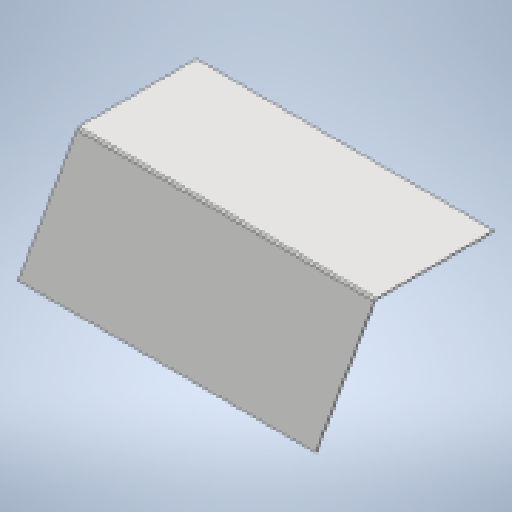
# Autodesk Inventor part: TRM 017 sheet in
Saved by Autodesk Inventor 2025 (Build 290162010, 162A)
## iProperties
Created: 2024-08-07
Part Number: TRM 017 sheet in
Material: AISI 304
Document SubType Name: Sheet Metal
Designer: pokla
Density: 8.02768 g/cm^3
Flat Pattern Width: 50 cm
Flat Pattern Length: 77.1162 cm
Flat Pattern Area: 3855.81 cm^2
Sheet Metal Rule: AISI304 2mm Die16
Sheet Metal Width: 500,000 mm
Sheet Metal Length: 771,162 mm
Sheet Metal Area: 385580,927 mm^2
Appearance: Default
Author: pokla
Autodesk Inventor part; units mm, degrees
ref_plane "YZ Plane" through (0, 0, 0) normal (1, 0, 0) x (0, 1, 0)
ref_plane "XZ Plane" through (0, 0, 0) normal (0, 1, 0) x (-1, 0, 0)
ref_plane "XY Plane" through (0, 0, 0) normal (0, 0, 1) x (1, 0, 0)
sketch "Sketch1" plane through (0, 0, 0) normal (0, 0, 1) x (1, 0, 0)
  line L0 (-250, -25) -> (250, -25)
  line L1 (250, -25) -> (250, 25)
  line L2 (250, 25) -> (-250, 25)
  line L3 (-250, 25) -> (-250, -25)
  line L4 (-250, -25) -> (250, 25) construction
  line L5 (250, -25) -> (-250, 25) construction
  point P0 (0, 0)
  dimension "d0" = 500
  dimension "d1" = 50
  measures "d0" distance of L2.end L1.end
  measures "d1" distance of L1.end L0.end
extrude "Plate1" add sketch "Sketch1" along normal blind 2
sketch "Sketch2" plane through (0, 0, 0) normal (0, 0, -1) x (-1, 0, 0)
  line L0 (-230, 5) -> (-30, 5) construction
  line L1 (-30, 5) -> (-30, -15) construction
  line L2 (-30, -15) -> (-230, -15) construction
  line L3 (-230, -15) -> (-230, 5) construction
  line L4 (-250, 25) -> (250, 25) projected
  line L5 (-250, -25) -> (-250, 25) projected
  point P0 (0, 0)
  point P1 (-48, 100)
  point P2 (250, 25)
  point P3 (-50, 98)
  dimension "d6" = 200
  dimension "d9" = 20
  dimension "d10" = 20
  dimension "d11" = 20
  constraints: 4 other
  measures "d6" distance of L0.start L0.end
  measures "d9" distance of L0.end L1.end
  measures "d11" length of L3
mark "Mark1"
sketch "Sketch3" plane through (-250, -23.1206, 1.316) normal (0, -0.9396926, 0.3420201) x (1, 0, 0)
  line L0 (500, 0) -> (0, 0)
  line L1 (0, 0) -> (0, -400)
  line L2 (0, -400) -> (500, -400)
  line L3 (500, -400) -> (500, 0)
  constraints: 6 end point, 1 horizontal, 1 perpendicular, 1 vertical
edge flange "Flange1" height 400 angle 70 thickness 2 bend radius 2.75 thickness toward (0, -0.9396926, 0.3420201) relief round relief width 2 relief depth 1 edges at (0, -25, 0) wall of the first edge with corners at (250, -23.1206, 1.316) (-250, -23.1206, 1.316) (-250, -159.9287, -374.5611) (250, -159.9287, -374.5611)
bend "Bend1"
corner "Corner1"
sketch "Sketch4" plane through (250, -159.9287, -372.5611) normal (0, 0, -1) x (-1, 0, 0)
  line L0 (500, 0) -> (0, 0)
  line L1 (0, 0) -> (0, -180)
  line L2 (0, -180) -> (500, -180)
  line L3 (500, -180) -> (500, 0)
  constraints: 6 end point, 1 horizontal, 1 perpendicular, 1 vertical
edge flange "Flange2" height 180 angle 70 thickness 2 bend radius 2.75 thickness toward (0, 0, -1) relief round relief width 2 relief depth 1 edges at (0, -161.8081, -373.877) wall of the first edge with corners at (-250, -159.9287, -372.5611) (250, -159.9287, -372.5611) (250, -339.9287, -372.5611) (-250, -339.9287, -372.5611)
bend "Bend2"
corner "Corner2"
sketch "Sketch5" plane through (250, -338.5145, -373.1469) normal (0, -0.7071068, -0.7071068) x (1, 0, 0)
  line L0 (-500, 0) -> (0, 0)
  line L1 (0, 0) -> (0, 100)
  line L2 (0, 100) -> (-500, 100)
  line L3 (-500, 100) -> (-500, 0)
  constraints: 6 end point, 1 horizontal, 1 perpendicular, 1 vertical
edge flange "Flange3" height 100 angle 45 thickness 2 bend radius 2.75 thickness toward (0, -0.7071068, -0.7071068) relief round relief width 2 relief depth 1 edges at (0, -339.9287, -372.5611) wall of the first edge with corners at (-250, -338.5145, -373.1469) (250, -338.5145, -373.1469) (250, -409.2251, -302.4362) (-250, -409.2251, -302.4362)
bend "Bend3"
corner "Corner3"
sketch "Sketch6" plane through (-250, -407.9396, -303.9683) normal (0, -0.6427876, 0.7660444) x (1, 0, 0)
  line L0 (500, 0) -> (0, 0)
  line L1 (0, 0) -> (0, -50)
  line L2 (0, -50) -> (500, -50)
  line L3 (500, -50) -> (500, 0)
  constraints: 6 end point, 1 horizontal, 1 perpendicular, 1 vertical
edge flange "Flange4" height 50 angle 85 thickness 2 bend radius 2.75 thickness toward (0, -0.6427876, 0.7660444) relief round relief width 2 relief depth 1 edges at (0, -410.6394, -303.8504) wall of the first edge with corners at (250, -407.9396, -303.9683) (-250, -407.9396, -303.9683) (-250, -446.2418, -336.1077) (250, -446.2418, -336.1077)
bend "Bend4"
corner "Corner4"
equation "\"d2\" = Thickness"
equation "\"d12\" = BendReliefWidth"
equation "\"d13\" = BendReliefDepth"
equation "\"d14\" = MinimumRemnant"
equation "\"d15\" = TransitionRadius"
equation "\"d18\" = BendRadius"
equation "\"d19\" = CornerReliefSize"
equation "\"d20\" = GapSize"
equation "\"d21\" = JacobiRadiusSize"
equation "\"d22\" = BendReliefWidth"
equation "\"d23\" = BendReliefDepth"
equation "\"d24\" = MinimumRemnant"
equation "\"d25\" = TransitionRadius"
equation "\"d28\" = BendRadius"
equation "\"d29\" = CornerReliefSize"
equation "\"d30\" = GapSize"
equation "\"d31\" = JacobiRadiusSize"
equation "\"d32\" = BendReliefWidth"
equation "\"d33\" = BendReliefDepth"
equation "\"d34\" = MinimumRemnant"
equation "\"d35\" = TransitionRadius"
equation "\"d38\" = BendRadius"
equation "\"d39\" = CornerReliefSize"
equation "\"d40\" = GapSize"
equation "\"d41\" = JacobiRadiusSize"
equation "\"d42\" = BendReliefWidth"
equation "\"d43\" = BendReliefDepth"
equation "\"d44\" = MinimumRemnant"
equation "\"d45\" = TransitionRadius"
equation "\"d48\" = BendRadius"
equation "\"d49\" = CornerReliefSize"
equation "\"d50\" = GapSize"
equation "\"d51\" = JacobiRadiusSize"
equation "\"BendReliefWidth\" = Thickness"
equation "\"BendReliefDepth\" = 0.5 * Thickness"
equation "\"CornerReliefSize\" = 4 * Thickness"
equation "\"MinimumRemnant\" = 2 * Thickness"
equation "\"TransitionRadius\" = BendRadius"
equation "\"JacobiRadiusSize\" = BendRadius"
equation "\"GapSize\" = Thickness"
equation "\"Thickness\" = 2"
equation "\"BendRadius\" = 2.75"
body "Solid1"
